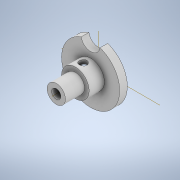
# Autodesk Inventor part: Деталь1
Saved by Autodesk Inventor 2021 (Build 250183000, 183)
## iProperties
Created: 2020-05-28
Part Number: Деталь1
Material: Типовые
Document SubType Name: Modeling
Designer: 2000
Density: 1 g/cm^3
Appearance: По умолчанию
Author: 2000
Autodesk Inventor part; units mm, degrees
ref_plane "YZ Plane" through (0, 0, 0) normal (1, 0, 0) x (0, 1, 0)
ref_plane "XZ Plane" through (0, 0, 0) normal (0, 1, 0) x (-1, 0, 0)
ref_plane "XY Plane" through (0, 0, 0) normal (0, 0, 1) x (1, 0, 0)
sketch "Эскиз1" plane through (0, 0, 0) normal (0, 0, 1) x (1, 0, 0)
  circle A0 centre (0, 0) radius 38
  circle A1 centre (0, 0) radius 13
  dimension "d0" = 76
  dimension "d1" = 26
  constraints: 2 centre point, 2 coincident
  measures "d0" diameter of A0
  measures "d1" diameter of A1
extrude "Выдавливание1" add sketch "Эскиз1" along normal blind 10
sketch "Эскиз2" plane through (0, 0, 10) normal (0, 0, 1) x (1, 0, 0)
  circle A0 centre (0, 0) radius 38 projected
  circle A1 centre (0, 38) radius 12.5
  point P0 (12.3298, 35.9441)
  point P1 (-12.3298, 35.9441)
  dimension "d10" = 25
  constraints: 1 centre point, 2 other
  measures "d10" diameter of A1
chamfer "Фаска1" distance 10 angle 45 1 edges at (-13, 0, 0)
sketch "Эскиз3" plane through (0, 0, 10) normal (0, 0, 1) x (1, 0, 0)
  circle A0 centre (0, 0) radius 18
  dimension "d18" = 36
  constraints: 1 centre point, 1 coincident
  measures "d18" diameter of A0
extrude "Выдавливание3" cut sketch "Эскиз2" against normal blind 10 contours A1 A0 | A0 A1 picked at (0, 33.6798) picked at (-0.3438, 41.9989)
extrude "Выдавливание4" add sketch "Эскиз3" along normal blind 20
sketch "Эскиз4" plane through (0, 0, 30) normal (0, 0, 1) x (1, 0, 0)
  circle A0 centre (0, 0) radius 12
  dimension "d17" = 24
  constraints: 1 centre point, 1 coincident
  measures "d17" diameter of A0
extrude "Выдавливание5" add sketch "Эскиз4" along normal blind 25
sketch "Эскиз5" plane through (0, 0, 0) normal (0, 1, 0) x (-1, 0, 0)
  circle A0 centre (0, 20) radius 5
  line L0 (12, 55) -> (-12, 55) projected
  point P0 (0, 0)
  dimension "d21" = 35
  dimension "d22" = 10
  constraints: 1 centre point
  measures "d21" distance from line of L0 A0.centre
  measures "d22" diameter of A0
extrude "Выдавливание6" cut sketch "Эскиз5" along normal blind 25
sketch "Эскиз6" plane through (0, 0, 30) normal (0, 0, 1) x (1, 0, 0)
  point P0 (0, 0)
sketch "Эскиз7" plane through (0, 0, 10) normal (0, 0, -1) x (-1, 0, 0)
  point P0 (0, 0)
sketch "Эскиз8" plane through (0, 0, 55) normal (0, 0, 1) x (1, 0, 0)
  circle A0 centre (0, 0) radius 6
  dimension "d25" = 12
  constraints: 1 centre point, 1 coincident
  measures "d25" diameter of A0
extrude "Выдавливание7" cut sketch "Эскиз8" against normal blind 28
sketch "Эскиз9" plane through (0, 0, 10) normal (0, 0, -1) x (-1, 0, 0)
  circle A0 centre (0, 0) radius 13
  dimension "d28" = 26
  constraints: 1 centre point, 1 coincident
  measures "d28" diameter of A0
extrude "Выдавливание8" cut sketch "Эскиз9" against normal blind 17
sketch "Эскиз10" plane through (0, 0, 0) normal (0, 1, 0) x (-1, 0, 0)
  point P0 (0, 0)
